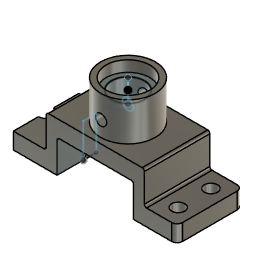
practice_4 v3 (Autodesk Fusion 360 design; units mm, degrees)
Autodesk Fusion 360 part; units mm, degrees
sketch "Sketch2" plane through (0, 0, 0) normal (0, 0, 1) x (1, 0, 0)
  line L0 (-75, 30) -> (75, 30)
  line L1 (75, 30) -> (75, -30)
  line L2 (75, -30) -> (-75, -30)
  line L3 (-75, -30) -> (-75, 30)
  point P0 (-75, 0)
  point P1 (0, 30)
  point P2 (-75, 30)
  point P3 (0, -30)
  point P4 (-75, -30)
  point P5 (-75, 0)
  point P6 (75, 0)
  point P7 (75, 80)
  point P8 (-75, 80)
  point P9 (75, 30)
  point P10 (-75, 30)
  point P11 (-75, -30)
  point P12 (75, -30)
  point P13 (-45, 30)
  point P14 (-45, -30)
  point P15 (75, -30)
  point P16 (75, 30)
  point P17 (45, 45)
  point P18 (-45, 45)
  point P19 (-45, 15)
  point P20 (-75, 15)
  point P21 (-75, 0)
  point P22 (-35, 0)
  point P23 (-35, 30)
  point P24 (35, 30)
  point P25 (35, 0)
  point P26 (75, 0)
  point P27 (75, 15)
  point P28 (45, 15)
  point P29 (-75, 30)
  point P30 (-75, -30)
  point P31 (75, -30)
  point P32 (75, 30)
  point P33 (30, 28)
  point P34 (-30, 28)
  point P35 (-30, 0)
  point P36 (30, 0)
  point P37 (-35, 31)
  point P38 (-35, 0)
  point P39 (-20, 0)
  point P40 (-20, 31)
  point P41 (30, 28)
  point P42 (-30, 28)
  point P43 (-30, 0)
  point P44 (30, 0)
  dimension "d3" = 150
  constraint horizontal L0
  constraint vertical L1
  constraint horizontal L2
  constraint vertical L3
  constraint coincident P29 P10
  measures "d3" distance of P29 P32
extrude "Extrude1" add sketch "Sketch2" along normal blind 80 makes body 1
sketch "Sketch3" plane through (0, 30, 0) normal (0, 1, 0) x (-1, 0, 0)
  line L0 (-75, 0) -> (75, 0)
  line L1 (75, 0) -> (75, 80)
  line L2 (75, 80) -> (-75, 80)
  line L3 (-75, 80) -> (-75, 0)
  line L4 (-35, 0) -> (35, 0)
  line L5 (35, 0) -> (35, 30)
  line L6 (35, 30) -> (-35, 30)
  line L7 (-35, 30) -> (-35, 0)
  point P0 (-35, 0)
  point P1 (35, 0)
  dimension "d6" = 30
  constraint coincident L0 P0
  constraint coincident L0 P1
  constraint horizontal L4
  constraint vertical L5
  constraint horizontal L6
  constraint vertical L7
  constraint coincident P0 L4.start
  measures "d6" distance of P0 L6.end
extrude "Extrude2" cut sketch "Sketch3" against normal blind 95 contours L0 L4 L5 L6 L7 bodies 1
sketch "Sketch4" plane through (0, 0, 80) normal (0, 0, 1) x (-1, 0, 0)
  line L0 (75, 30) -> (-75, 30)
  line L1 (-75, 30) -> (-75, -30)
  line L2 (-75, -30) -> (75, -30)
  line L3 (75, -30) -> (75, 30)
  line L4 (-75, 30) -> (-45, 30)
  line L5 (-45, 30) -> (-45, -30)
  line L6 (-45, -30) -> (-75, -30)
  line L7 (-75, -30) -> (-75, 30)
  dimension "d9" = 30
  dimension "d10" = 60
  constraint horizontal L4
  constraint vertical L5
  constraint horizontal L6
  constraint vertical L7
  constraint coincident L0.end L1.start
  measures "d9" distance of L0.end L4.end
  measures "d10" distance of L0.end L1.end
extrude "Extrude3" cut sketch "Sketch4" against normal blind 65 contours L0 L1 L2 L4 L5 L6 L7 bodies 1
sketch "Sketch5" plane through (0, 0, 80) normal (0, 0, 1) x (-1, 0, 0)
  line L0 (-45, 30) -> (-45, -30)
  line L1 (-45, -30) -> (75, -30)
  line L2 (75, -30) -> (75, 30)
  line L3 (75, 30) -> (-45, 30)
  line L4 (45, 30) -> (75, 30)
  line L5 (75, 30) -> (75, -30)
  line L6 (75, -30) -> (45, -30)
  line L7 (45, -30) -> (45, 30)
  constraint horizontal L4
  constraint vertical L5
  constraint horizontal L6
  constraint vertical L7
  constraint coincident L1.end L2.start
  constraint coincident L3 L4.start
extrude "Extrude4" cut sketch "Sketch5" against normal blind 65 contours L1 L2 L3 L4 L5 L6 L7 bodies 1
extrude "Extrude5" cut 1 faces at (-15, 10, 80) along direction (0, 0, -1) blind 35 on bodies 1 bodies 1
sketch "Sketch6" plane through (0, 30, 0) normal (0, 1, 0) x (-1, 0, 0)
  line L0 (45, 45) -> (-45, 45)
  line L1 (-45, 45) -> (-45, 15)
  line L2 (-45, 15) -> (-75, 15)
  line L3 (-75, 15) -> (-75, 0)
  line L4 (-75, 0) -> (-35, 0)
  line L5 (-35, 0) -> (-35, 30)
  line L6 (-35, 30) -> (35, 30)
  line L7 (35, 30) -> (35, 0)
  line L8 (35, 0) -> (75, 0)
  line L9 (75, 0) -> (75, 15)
  line L10 (75, 15) -> (45, 15)
  line L11 (45, 15) -> (45, 45)
sketch "Sketch7" plane through (0, 30, 0) normal (0, 1, 0) x (-1, 0, 0)
fillet "Fillet1" radius 2 1 edges at (-45, 0, 45) on bodies 1
fillet "Fillet2" radius 2 1 edges at (45, 0, 45) on bodies 1
fillet "Fillet3" radius 2 1 edges at (45, 0, 15) on bodies 1
fillet "Fillet4" radius 2 1 edges at (-45, 0, 15) on bodies 1
sketch "Sketch8" plane through (0, 0, 15) normal (0, 0, 1) x (-1, 0, 0)
  line L0 (-47, -30) -> (-47, 30)
  line L1 (-47, 30) -> (-75, 30)
  line L2 (-75, 30) -> (-75, -30)
  line L3 (-75, -30) -> (-47, -30)
  line L4 (-61, 30) -> (-61, -30)
  line L5 (-75, 0) -> (-47, 0)
  circle A0 centre (-61, 15) radius 6
  circle A1 centre (-61, -15) radius 6
  dimension "d25" = 12
  dimension "d26" = 12
  constraint midpoint L1 L4.start
  constraint midpoint L3 L4.end
  constraint midpoint L2 L5.start
  constraint midpoint L0 L5.end
  constraint coincident L4 A0.centre
  constraint coincident L4 A1.centre
  measures "d25" diameter of A0
  measures "d26" diameter of A1
extrude "Extrude6" cut sketch "Sketch8" against normal blind 14 contours L4 A1 | L4 A1 bodies 1
extrude "Extrude7" cut 1 faces at (59.4674, 14.5272, 1) along direction (0, 0, -1) blind 16 on bodies 1 bodies 1
extrude "Extrude8" cut sketch "Sketch8" against normal blind 21 contours L4 A0 | L4 A0 bodies 1
sketch "Sketch9" plane through (0, 0, 15) normal (0, 0, 1) x (-1, 0, 0)
  line L0 (47, 30) -> (47, -30)
  line L1 (47, -30) -> (75, -30)
  line L2 (75, -30) -> (75, 30)
  line L3 (75, 30) -> (47, 30)
  circle A0 centre (75, 0) radius 7
  dimension "d33" = 14
  constraint midpoint L2 A0.centre
  measures "d33" diameter of A0
extrude "Extrude9" cut sketch "Sketch9" against normal blind 34 contours L2 A0 picked at (72.7252, 0.5192) bodies 1
sketch "Sketch10" plane through (0, 0, 15) normal (0, 0, 1) x (-1, 0, 0)
  circle A0 centre (-70, 25) radius 5
  circle A1 centre (-70, -25) radius 5
  arc A2 (-75, -25) -> (-70, -30) centre (-72.5, -27.5) ccw
  arc A3 (-70, 30) -> (-75, 25) centre (-72.5, 27.5) ccw
  point P0 (-72.5, 30)
  point P1 (-75, 27.5)
  point P2 (-75, 30)
  point P3 (-70, 30)
  point P4 (-75, 25)
  point P5 (-70, -30)
  point P6 (-75, -25)
  dimension "d37" = 10
  dimension "d38" = 10
  constraint coincident A0 P3
  constraint coincident A0 P4
  constraint coincident A1 P5
  constraint coincident P6 A2.start
  constraint coincident P5 A2.end
  constraint coincident P2 A3
  constraint coincident P4 A3.end
  constraint coincident P3 A3.start
  measures "d37" diameter of A0
  measures "d38" diameter of A1
extrude "Extrude10" cut sketch "Sketch10" against normal blind 17 contours A0 A3 bodies 1
extrude "Extrude11" cut sketch "Sketch10" against normal blind 23 contours A1 A2 bodies 1
sketch "Sketch11" plane through (0, 0, 45) normal (0, 0, 1) x (-1, 0, 0)
  line L0 (-43, 30) -> (-43, -30)
  line L1 (-43, -30) -> (43, -30)
  line L2 (43, -30) -> (43, 30)
  line L3 (43, 30) -> (-43, 30)
sketch "Sketch12" plane through (0, 0, 45) normal (0, 0, 1) x (-1, 0, 0)
sketch "Sketch13" plane through (0, 0, 45) normal (0, 0, 1) x (-1, 0, 0)
  circle A0 centre (0, 0) radius 25
  point P0 (0, 30)
  point P1 (75, 30)
  point P2 (0, -30)
  point P3 (-45, 0)
  point P4 (47, 0)
  dimension "d43" = 50
  constraint coincident A0.centre origin
  measures "d43" diameter of A0
extrude "Extrude12" add sketch "Sketch13" along normal blind 35 bodies 1
sketch "Sketch14" plane through (0, 0, 80) normal (0, 0, 1) x (-1, 0, 0)
  circle A0 centre (0, 0) radius 25
  circle A1 centre (0, 0) radius 20
  dimension "d46" = 40
  constraint concentric A0 A1
  measures "d46" diameter of A1
extrude "Extrude13" cut sketch "Sketch14" against normal blind 10 contours A1 bodies 1
sketch "Sketch15" plane through (0, 0, 70) normal (0, 0, 1) x (-1, 0, 0)
  circle A0 centre (0, 0) radius 20
  circle A1 centre (0, 0) radius 15
  dimension "d49" = 30
  constraint coincident A0.centre A1.centre
  measures "d49" diameter of A1
extrude "Extrude14" cut sketch "Sketch15" against normal blind 25 contours A1 bodies 1
sketch "Sketch16" plane through (0, 0, 0) normal (0, 1, 0) x (1, 0, 0)
  line L0 (0, -80) -> (0, -59)
  circle A0 centre (0, -59) radius 5
  point P0 (0, -80)
  dimension "d52" = 21
  dimension "d53" = 10
  constraint coincident P0 L0.start
  constraint vertical L0
  constraint coincident L0.end A0.centre
  measures "d52" distance of P0 L0.end
  measures "d53" diameter of A0
extrude "Extrude15" cut sketch "Sketch16" along normal blind -40 and the other way blind -40 bodies 1
fillet "Fillet5" radius 2 1 edges at (-35, 0, 30) on bodies 1
fillet "Fillet6" radius 2 1 edges at (35, 0, 30) on bodies 1
sketch "Sketch17" plane through (-35, 0, 0) normal (1, 0, 0) x (0, 1, 0)
  line L0 (30, 28) -> (-30, 28)
  line L1 (-30, 28) -> (-30, 0)
  line L2 (-30, 0) -> (30, 0)
  line L3 (30, 0) -> (30, 28)
  line L4 (-6, 0) -> (6, 0)
  line L5 (-6, 0) -> (-6, 31)
  line L6 (-6, 31) -> (6, 31)
  line L7 (6, 31) -> (6, 0)
  constraint coincident L2 L4.start
  constraint coincident L2 L4.end
  constraint perpendicular L0 L5
  constraint perpendicular L5 L6
  constraint perpendicular L2 L7
extrude "Extrude16" add sketch "Sketch17" along normal blind 15 separate body contours L0 L2 L4 L5 L7 | L0 L5 L6 L7 makes body 2
sketch "Sketch18" plane through (0, -6, 0) normal (0, -1, 0) x (1, 0, 0)
  line L0 (-35, 31) -> (-35, 0)
  line L1 (-35, 0) -> (-20, 0)
  line L2 (-20, 0) -> (-20, 31)
  line L3 (-20, 31) -> (-35, 31)
  line L4 (-35, 0) -> (-20, 30)
  line L5 (-35, 0) -> (-20, 0)
  line L6 (-20, 0) -> (-20, 30)
  constraint coincident L0.end L1.start
  constraint coincident L2 L4.end
  constraint coincident L1.end L2.start
extrude "Extrude17" cut sketch "Sketch18" against normal blind 54 contours L1 L2 L4 L5 L6 bodies 2
sketch "Sketch19" plane through (35, 0, 0) normal (-1, 0, 0) x (0, -1, 0)
  line L0 (30, 28) -> (-30, 28)
  line L1 (-30, 28) -> (-30, 0)
  line L2 (-30, 0) -> (30, 0)
  line L3 (30, 0) -> (30, 28)
copy_body "CopyPasteBodies1" bodies 2 makes body 3
move_body "Move1" bodies 3 to x (-1, 0, 0) y (0, -1, 0) z (0, 0, 1) at (-27, -12, 0)
move_body "Move2" bodies 3 to x (1, 0, 0) y (0, 1, 0) z (0, 0, 1) at (27, 12, 0)
sketch "Sketch20" plane through (0, 0, 0) normal (0, 1, 0) x (1, 0, 0)
extrude "Extrude18" cut sketch "Sketch15" against normal blind 45 contours A1 bodies 1
combine "Combine1" operation add target body 1 tool bodies 2 3
